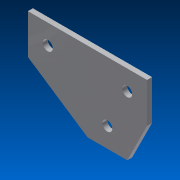
# Autodesk Inventor part: TriangleBracket
Saved by Autodesk Inventor 2013 (Build 170138000, 138)
## iProperties
Created: 2013-07-20
Part Number: TriangleBracket
Material: Aluminum 6061
Document SubType Name: Modeling
Designer: robotics
Density: 1 g/cm^3
Author: robotics
Autodesk Inventor part; units mm, degrees
ref_plane "YZ Plane" through (0, 0, 0) normal (1, 0, 0) x (0, 1, 0)
ref_plane "XZ Plane" through (0, 0, 0) normal (0, 1, 0) x (-1, 0, 0)
ref_plane "XY Plane" through (0, 0, 0) normal (0, 0, 1) x (1, 0, 0)
sketch "Sketch1" plane through (0, 0, 0) normal (0, 0, 1) x (1, 0, 0)
  line L0 (0, 0) -> (0, 25.4)
  line L1 (0, 25.4) -> (76.2, 25.4)
  line L2 (76.2, 25.4) -> (76.2, 0)
  line L3 (76.2, 0) -> (63.5, -25.4)
  line L4 (63.5, -25.4) -> (38.1, -25.4)
  line L5 (38.1, -25.4) -> (0, 0)
  dimension "d1" = 25.4
  dimension "d2" = 25.4
  dimension "d3" = 25.4
  dimension "d4" = 76.2
  dimension "d5" = 50.8
  dimension "d6" = 38.1
  constraints: 12 end point, 1 parallel, 1 perpendicular, 1 vertical
  measures "d1" distance of L0.start L0.end
  measures "d2" distance of L1.end L2.end
  measures "d3" distance of L3.end L4.end
  measures "d4" distance of L0.end L1.end
  measures "d5" distance between parallel lines of L4 L1
  measures "d6" distance from line of L0 L4.end
extrude "Extrusion1" add sketch "Sketch1" along normal blind 3.175
sketch "Sketch2" plane through (0, 0, 3.175) normal (0, 0, 1) x (1, 0, 0)
  line L0 (0, 25.4) -> (0, 0) projected
  line L1 (38.1, -25.4) -> (63.5, -25.4) projected
  line L2 (76.2, -25.4) -> (76.2, 25.4) projected
  line L3 (76.2, 25.4) -> (0, 25.4) projected
  point P0 (76.2, 0)
  point P1 (12.7, 12.7)
  point P2 (63.5, 12.7)
  point P3 (50.8, -12.7)
  dimension "d9" = 12.7
  dimension "d10" = 12.7
  dimension "d11" = 12.7
  dimension "d12" = 12.7
  dimension "d13" = 12.7
  dimension "d14" = 12.7
  dimension "d22" = 52.3634
  constraints: 1 other
  measures "d9" distance from line of L3 point (12.7, 12.7)
  measures "d10" distance from line of L0 point (12.7, 12.7)
  measures "d11" distance from line of point (63.5, 12.7) L3
  measures "d13" distance from line of L1 point (50.8, -12.7)
  measures "d14" horizontal distance of L1.end point (50.8, -12.7)
  measures "d22" distance of L1.end L3.start
hole "Hole1" at (12.7, 12.7, 3.175) at (63.5, 12.7, 3.175) at (50.8, -12.7, 3.175) direction (0, 0, -1) diameter 6.35 end through all
body "Solid1"
